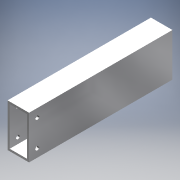
# Autodesk Inventor part: SupportExtrusion
Saved by Autodesk Inventor 2019.4 (Build 234330000, 330)
## iProperties
Created: 2019-12-31
Part Number: SupportExtrusion
Material: Aluminum 6061
Document SubType Name: Modeling
Designer: Mark
Mass: 272.16 g
Surface Area: 682.08 cm^2
Volume: 100.8 cm^3
Density: 2.7 g/cm^3
Appearance: Aluminum - Flat
Author: Mark
Autodesk Inventor part; units mm, degrees
ref_plane "YZ Plane" through (0, 0, 0) normal (1, 0, 0) x (0, 1, 0)
ref_plane "XZ Plane" through (0, 0, 0) normal (0, 1, 0) x (-1, 0, 0)
ref_plane "XY Plane" through (0, 0, 0) normal (0, 0, 1) x (1, 0, 0)
sketch "Sketch1" plane through (0, 0, 0) normal (0, 0, 1) x (1, 0, 0)
  line L0 (-15, -30) -> (15, -30)
  line L1 (15, -30) -> (15, 30)
  line L2 (15, 30) -> (-15, 30)
  line L3 (-15, 30) -> (-15, -30)
  line L4 (-15, -30) -> (15, 30) construction
  line L5 (15, -30) -> (-15, 30) construction
  line L6 (-12, -27) -> (12, -27)
  line L7 (12, -27) -> (12, 27)
  line L8 (12, 27) -> (-12, 27)
  line L9 (-12, 27) -> (-12, -27)
  line L10 (-12, -27) -> (12, 27) construction
  line L11 (12, -27) -> (-12, 27) construction
  point P0 (0, 0)
  dimension "d0" = 30
  dimension "d1" = 60
  dimension "d2" = 24
  dimension "d3" = 54
  constraints: 24 end point, 4 midpoint, 4 parallel, 2 horizontal, 2 perpendicular
  measures "d0" distance of L2.end L1.end
  measures "d1" distance of L1.end L0.end
  measures "d2" distance of L8.end L7.end
  measures "d3" distance of L7.end L6.end
extrude "Extrusion1" add sketch "Sketch1" along normal blind 200
sketch "Sketch2" plane through (-15, -30, 0) normal (-1, 0, 0) x (0, 0, 1)
  circle A0 centre (188.5, 50) radius 2.75
  circle A1 centre (188.5, 10) radius 2.75
  line L0 (200, 60) -> (200, 0) projected
  line L1 (0, 0) -> (200, 0) projected
  line L2 (0, 60) -> (200, 60) projected
  point P0 (0, 30)
  dimension "d6" = 5.5
  dimension "d7" = 5.5
  dimension "d8" = 11.5
  dimension "d9" = 10
  dimension "d10" = 11.5
  dimension "d11" = 10
  constraints: 2 centre point
  measures "d6" diameter of A0
  measures "d7" diameter of A1
  measures "d8" distance from line of L0 A1.centre
  measures "d9" distance from line of L1 A1.centre
  measures "d10" distance from line of L0 A0.centre
  measures "d11" distance from line of L2 A0.centre
extrude "Extrusion2" cut sketch "Sketch2" against normal blind 30
body "Solid1"
